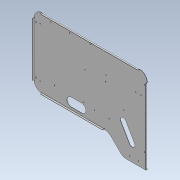
# Autodesk Inventor part: Монтажный лист
Saved by Autodesk Inventor 2021.2 (Build 252289000, 289)
## iProperties
Created: 2022-11-29
Part Number: Монтажный лист
Material: Типовые
Document SubType Name: ЛистМат
Designer: Voodoo
Density: 1 g/cm^3
Sheet Metal Rule: По умолчанию_мм
Appearance: По умолчанию
Mass: 97.8179 g
Surface Area: 1975.67 cm^2
Volume: 97.8179 cm^3
Flat Pattern Width: 29.2262 cm
Flat Pattern Length: 39.5524 cm
Flat Pattern Area: 1155.97 cm^2
Sheet Metal Width: 292,262 мм
Sheet Metal Length: 395,524 мм
Sheet Metal Area: 115596,583 мм^2
Author: Voodoo
Autodesk Inventor part; units mm, degrees
ref_plane "YZ Plane" through (0, 0, 0) normal (1, 0, 0) x (0, 1, 0)
ref_plane "XZ Plane" through (0, 0, 0) normal (0, 1, 0) x (-1, 0, 0)
ref_plane "XY Plane" through (0, 0, 0) normal (0, 0, 1) x (1, 0, 0)
sketch "Эскиз1" plane through (0, 0, 0) normal (0, 0, 1) x (1, 0, 0)
  line L0 (-166.5, -124) -> (46.0736, -124)
  line L1 (198.5, -124) -> (198.5, 92)
  line L2 (166.5, 124) -> (-166.5, 124)
  line L3 (-198.5, 92) -> (-198.5, -92)
  line L4 (-198.5, -124) -> (198.5, 124) construction
  line L5 (198.5, -124) -> (-198.5, 124) construction
  arc A0 (-166.5, 124) -> (-198.5, 92) centre (-166.5, 92) ccw
  arc A1 (198.5, 92) -> (166.5, 124) centre (166.5, 92) ccw
  arc A2 (-198.5, -92) -> (-166.5, -124) centre (-166.5, -92) ccw
  line L6 (198.5, -124) -> (198.5, -162)
  line L7 (186.5, -174) -> (120.9264, -174)
  line L8 (99.7132, -165.2132) -> (67.2868, -132.7868)
  arc A3 (186.5, -174) -> (198.5, -162) centre (186.5, -162) ccw
  arc A4 (99.7132, -165.2132) -> (120.9264, -174) centre (120.9264, -144) ccw
  arc A5 (67.2868, -132.7868) -> (46.0736, -124) centre (46.0736, -154) ccw
  line L9 (-166.5, 119) -> (166.5, 119)
  arc A6 (193.5, 92) -> (166.5, 119) centre (166.5, 92) ccw
  line L10 (193.5, 92) -> (193.5, -145)
  line L11 (193.5, -145) -> (193.5, -162)
  arc A7 (186.5, -169) -> (193.5, -162) centre (186.5, -162) ccw
  line L12 (186.5, -169) -> (120.9264, -169)
  arc A8 (103.2487, -161.6777) -> (120.9264, -169) centre (120.9264, -144) ccw
  line L13 (103.2487, -161.6777) -> (70.8223, -129.2513)
  arc A9 (70.8223, -129.2513) -> (46.0736, -119) centre (46.0736, -154) ccw
  line L14 (46.0736, -119) -> (-166.5, -119)
  arc A10 (-193.5, -92) -> (-166.5, -119) centre (-166.5, -92) ccw
  line L15 (-193.5, -92) -> (-193.5, 92)
  arc A11 (-166.5, 119) -> (-193.5, 92) centre (-166.5, 92) ccw
  point P0 (0, 0)
  point P1 (198.5, -174)
  point P2 (108.5, -174)
  dimension "d2" = 397
  dimension "d3" = 248
  dimension "d4" = 32
  dimension "d5" = 298
  dimension "d6" = 12
  dimension "d7" = 50
  dimension "d8" = 90
  dimension "d9" = 135
  dimension "d10" = 30
  dimension "d11" = 5
  constraints: 32 end point, 24 point on circle, 12 centre point, 12 point on line, 12 tangent, 4 parallel, 4 perpendicular, 3 equal radius, 2 midpoint, 1 horizontal, 12 other
  measures "d2" distance of L5.end L4.end
  measures "d3" distance of L4.end L1.start
  measures "d4" radius of A0
  measures "d5" distance between parallel lines of L7 L2
  measures "d6" radius of A3
  measures "d7" distance between parallel lines of L0 L7
  measures "d8" distance from line of L6 point (108.5, -174)
  measures "d9" angle of L0 L8
  measures "d10" radius of A4
  measures "d11" distance between parallel lines of L2 L9
extrude "Пластина1" add sketch "Эскиз1" along normal blind 1 contours L9 A6 L10 L11 A7 L12 A8 L13 A9 L14 A10 L15 A11
sketch "Эскиз4" plane through (-192.5, -92, 0) normal (-1, 0, 0) x (0, -1, 0)
  line L0 (-184, 0) -> (0, 0)
  line L1 (0, 0) -> (0, 6)
  line L2 (0, 6) -> (-184, 6)
  line L3 (-184, 6) -> (-184, 0)
  constraints: 6 end point, 1 horizontal, 1 perpendicular, 1 vertical
edge flange "Фланец1" height 6 angle 90 thickness 1 bend radius 1 thickness toward (-1, 0, 0) relief straight relief width 1 relief depth 0.5 corner gap 1 corner form 0 edges at (-193.5, 0, 1) (-60.2132, -119, 1) (0, 119, 1) (193.5, -26.5, 1) (193.5, -153.5, 1) wall of the first edge with corners at (-192.5, 92, 0) (-192.5, -92, 0) (-192.5, -92, 6) (-192.5, 92, 6)
bend "Сгиб1"
corner "УглСтык1"
sketch "Эскиз5" plane through (0, 0, 1) normal (0, 0, 1) x (1, 0, 0)
  arc A0 (-193.4815, -93) -> (-167.5, -118.9815) centre (-166.5, -92) ccw projected
  arc A1 (70.8223, -129.2513) -> (47.0736, -119.0143) centre (46.0736, -154) ccw projected
  line L0 (103.2487, -161.6777) -> (70.8223, -129.2513) projected
  arc A2 (103.2487, -161.6777) -> (120.9264, -169) centre (120.9264, -144) ccw projected
  line L1 (186.5, -169) -> (120.9264, -169) projected
  arc A3 (186.5, -169) -> (193.4282, -163) centre (186.5, -162) ccw projected
  arc A4 (193.4815, 93) -> (167.5, 118.9815) centre (166.5, 92) ccw projected
  arc A5 (-167.5, 118.9815) -> (-193.4815, 93) centre (-166.5, 92) ccw projected
  circle A6 centre (-186, 82) radius 2.5
  circle A7 centre (-186, -82) radius 2.5
  circle A8 centre (0, 111.1) radius 2.5
  circle A9 centre (185.8, 82) radius 2.5
  circle A10 centre (185.8, -116.8) radius 2.5
  line L2 (191, 93) -> (193.4815, 93) projected
  line L3 (167.5, 118.9815) -> (167.5, 116.5) projected
  line L4 (167.5, 116.5) -> (166.5, 116.5) projected
  line L5 (166.5, 116.5) -> (166.5, 117) projected
  line L6 (166.5, 117) -> (-166.5, 117) projected
  line L7 (-166.5, 117) -> (-166.5, 116.5) projected
  line L8 (-166.5, 116.5) -> (-167.5, 116.5) projected
  line L9 (-167.5, 116.5) -> (-167.5, 118.9815) projected
  line L10 (-193.4815, 93) -> (-191, 93) projected
  line L11 (-191, 93) -> (-191, 92) projected
  line L12 (-191, 92) -> (-191.5, 92) projected
  line L13 (-191.5, 92) -> (-191.5, -92) projected
  line L14 (-191.5, -92) -> (-191, -92) projected
  line L15 (-191, -92) -> (-191, -93) projected
  line L16 (-191, -93) -> (-193.4815, -93) projected
  line L17 (-167.5, -118.9815) -> (-167.5, -116.5) projected
  line L18 (-167.5, -116.5) -> (-166.5, -116.5) projected
  line L19 (-166.5, -116.5) -> (-166.5, -117) projected
  line L20 (-166.5, -117) -> (46.0736, -117) projected
  line L21 (46.0736, -117) -> (46.0736, -116.5) projected
  line L22 (46.0736, -116.5) -> (47.0736, -116.5) projected
  line L23 (47.0736, -116.5) -> (47.0736, -119.0143) projected
  line L24 (193.4282, -163) -> (191, -163) projected
  line L25 (191, -163) -> (191, -162) projected
  line L26 (191, -162) -> (191.5, -162) projected
  line L27 (191.5, -162) -> (191.5, 92) projected
  line L28 (191.5, 92) -> (191, 92) projected
  line L29 (191, 92) -> (191, 93) projected
  line L30 (166.5, 119) -> (-166.5, 119) projected
  line L31 (193.5, -162) -> (193.5, 92) projected
  line L32 (-193.5, 92) -> (-193.5, -92) projected
  line L33 (-166.5, -119) -> (46.0736, -119) projected
  point P0 (0, 0)
  point P1 (0, 119)
  dimension "d34" = 5
  dimension "d37" = 5
  dimension "d40" = 5
  dimension "d43" = 5
  dimension "d45" = 5
  dimension "d47" = 52.2
  dimension "d136" = 37
  dimension "d137" = 7.7
  dimension "d138" = 7.7
  dimension "d139" = 7.9
  dimension "d140" = 7.5
  dimension "d141" = 37
  dimension "d142" = 37
  dimension "d143" = 7.5
  constraints: 5 centre point, 1 midpoint, 1 vertical alignment
  measures "d34" diameter of A6
  measures "d37" diameter of A7
  measures "d40" diameter of A8
  measures "d43" diameter of A9
  measures "d45" diameter of A10
  measures "d47" distance from line of A10.centre L1
  measures "d136" distance from line of A9.centre L30
  measures "d137" distance from line of A10.centre L31
  measures "d138" distance from line of A9.centre L31
  measures "d139" distance from line of A8.centre L30
  measures "d140" distance from line of A6.centre L32
  measures "d141" distance from line of L30 A6.centre
  measures "d142" distance from line of L33 A7.centre
  measures "d143" distance from line of A7.centre L32
extrude "Вырез3" cut sketch "Эскиз5" against normal blind 1 contours A6 | A7 | A8 | A9 | A10
sketch "Эскиз6" plane through (0, 0, 1) normal (0, 0, 1) x (1, 0, 0)
  circle A0 centre (185.8, 82) radius 2.5 projected
  circle A1 centre (-186, -82) radius 2.5 projected
  circle A2 centre (-186, 82) radius 2.5 projected
  circle A3 centre (0, 111.1) radius 2.5 projected
  circle A4 centre (185.8, -116.8) radius 2.5 projected
  arc A5 (-193.4815, -93) -> (-167.5, -118.9815) centre (-166.5, -92) ccw projected
  arc A6 (70.8223, -129.2513) -> (47.0736, -119.0143) centre (46.0736, -154) ccw projected
  line L0 (103.2487, -161.6777) -> (70.8223, -129.2513) projected
  arc A7 (103.2487, -161.6777) -> (120.9264, -169) centre (120.9264, -144) ccw projected
  line L1 (186.5, -169) -> (120.9264, -169) projected
  arc A8 (186.5, -169) -> (193.4282, -163) centre (186.5, -162) ccw projected
  arc A9 (193.4815, 93) -> (167.5, 118.9815) centre (166.5, 92) ccw projected
  arc A10 (-167.5, 118.9815) -> (-193.4815, 93) centre (-166.5, 92) ccw projected
  circle A11 centre (-19.5, 24.5) radius 1.5
  circle A12 centre (51.5, 24.5) radius 1.5
  circle A13 centre (53, 44.5) radius 1.5
  circle A14 centre (154, 44.5) radius 1.5
  circle A15 centre (-135.8, 107) radius 1.5
  circle A16 centre (-71.5, 107) radius 1.5
  line L2 (191, 93) -> (193.4815, 93) projected
  line L3 (167.5, 118.9815) -> (167.5, 116.5) projected
  line L4 (167.5, 116.5) -> (166.5, 116.5) projected
  line L5 (166.5, 116.5) -> (166.5, 117) projected
  line L6 (166.5, 117) -> (-166.5, 117) projected
  line L7 (-166.5, 117) -> (-166.5, 116.5) projected
  line L8 (-166.5, 116.5) -> (-167.5, 116.5) projected
  line L9 (-167.5, 116.5) -> (-167.5, 118.9815) projected
  line L10 (-193.4815, 93) -> (-191, 93) projected
  line L11 (-191, 93) -> (-191, 92) projected
  line L12 (-191, 92) -> (-191.5, 92) projected
  line L13 (-191.5, 92) -> (-191.5, -92) projected
  line L14 (-191.5, -92) -> (-191, -92) projected
  line L15 (-191, -92) -> (-191, -93) projected
  line L16 (-191, -93) -> (-193.4815, -93) projected
  line L17 (-167.5, -118.9815) -> (-167.5, -116.5) projected
  line L18 (-167.5, -116.5) -> (-166.5, -116.5) projected
  line L19 (-166.5, -116.5) -> (-166.5, -117) projected
  line L20 (-166.5, -117) -> (46.0736, -117) projected
  line L21 (46.0736, -117) -> (46.0736, -116.5) projected
  line L22 (46.0736, -116.5) -> (47.0736, -116.5) projected
  line L23 (47.0736, -116.5) -> (47.0736, -119.0143) projected
  line L24 (193.4282, -163) -> (191, -163) projected
  line L25 (191, -163) -> (191, -162) projected
  line L26 (191, -162) -> (191.5, -162) projected
  line L27 (191.5, -162) -> (191.5, 92) projected
  line L28 (191.5, 92) -> (191, 92) projected
  line L29 (191, 92) -> (191, 93) projected
  line L30 (-193.5, 92) -> (-193.5, -92) projected
  line L31 (166.5, 119) -> (-166.5, 119) projected
  line L32 (193.5, -162) -> (193.5, 92) projected
  point P0 (0, 0)
  dimension "d51" = 3
  dimension "d52" = 3
  dimension "d53" = 3
  dimension "d54" = 3
  dimension "d56" = 71
  dimension "d58" = 101
  dimension "d61" = 3
  dimension "d62" = 3
  dimension "d63" = 64.3
  dimension "d123" = 74.5
  dimension "d124" = 39.5
  dimension "d125" = 142
  dimension "d126" = 20
  dimension "d127" = 12
  dimension "d128" = 122
  constraints: 6 centre point, 3 horizontal alignment
  measures "d51" diameter of A11
  measures "d52" diameter of A12
  measures "d53" diameter of A13
  measures "d54" diameter of A14
  measures "d56" distance of A12.centre A11.centre
  measures "d58" distance of A13.centre A14.centre
  measures "d61" diameter of A15
  measures "d62" diameter of A16
  measures "d63" distance of A16.centre A15.centre
  measures "d123" distance from line of L31 A14.centre
  measures "d124" distance from line of L32 A14.centre
  measures "d125" distance from line of L32 A12.centre
  measures "d126" vertical distance of A13.centre A12.centre
  measures "d127" distance from line of A16.centre L31
  measures "d128" distance from line of L30 A16.centre
extrude "Вырез4" cut sketch "Эскиз6" against normal blind 1 contours A11 | A12 | A13 | A14 | A15 | A16
sketch "Эскиз7" plane through (0, 0, 1) normal (0, 0, 1) x (1, 0, 0)
  circle A0 centre (-135.8, 107) radius 1.5 projected
  circle A1 centre (53, 44.5) radius 1.5 projected
  circle A2 centre (-19.5, 24.5) radius 1.5 projected
  circle A3 centre (51.5, 24.5) radius 1.5 projected
  circle A4 centre (154, 44.5) radius 1.5 projected
  circle A5 centre (-71.5, 107) radius 1.5 projected
  circle A6 centre (185.8, 82) radius 2.5 projected
  circle A7 centre (-186, -82) radius 2.5 projected
  circle A8 centre (-186, 82) radius 2.5 projected
  circle A9 centre (0, 111.1) radius 2.5 projected
  circle A10 centre (185.8, -116.8) radius 2.5 projected
  arc A11 (-193.4815, -93) -> (-167.5, -118.9815) centre (-166.5, -92) ccw projected
  arc A12 (70.8223, -129.2513) -> (47.0736, -119.0143) centre (46.0736, -154) ccw projected
  line L0 (103.2487, -161.6777) -> (70.8223, -129.2513) projected
  arc A13 (103.2487, -161.6777) -> (120.9264, -169) centre (120.9264, -144) ccw projected
  line L1 (186.5, -169) -> (120.9264, -169) projected
  arc A14 (186.5, -169) -> (193.4282, -163) centre (186.5, -162) ccw projected
  arc A15 (193.4815, 93) -> (167.5, 118.9815) centre (166.5, 92) ccw projected
  arc A16 (-167.5, 118.9815) -> (-193.4815, 93) centre (-166.5, 92) ccw projected
  circle A17 centre (-172.5, 84) radius 1.5
  circle A18 centre (-172.5, -86) radius 1.5
  circle A19 centre (172.5, 45) radius 1.5
  line L2 (0, 111.1) -> (0, 66.4707)
  line L3 (191, 93) -> (193.4815, 93) projected
  line L4 (167.5, 118.9815) -> (167.5, 116.5) projected
  line L5 (167.5, 116.5) -> (166.5, 116.5) projected
  line L6 (166.5, 116.5) -> (166.5, 117) projected
  line L7 (166.5, 117) -> (-166.5, 117) projected
  line L8 (-166.5, 117) -> (-166.5, 116.5) projected
  line L9 (-166.5, 116.5) -> (-167.5, 116.5) projected
  line L10 (-167.5, 116.5) -> (-167.5, 118.9815) projected
  line L11 (-193.4815, 93) -> (-191, 93) projected
  line L12 (-191, 93) -> (-191, 92) projected
  line L13 (-191, 92) -> (-191.5, 92) projected
  line L14 (-191.5, 92) -> (-191.5, -92) projected
  line L15 (-191.5, -92) -> (-191, -92) projected
  line L16 (-191, -92) -> (-191, -93) projected
  line L17 (-191, -93) -> (-193.4815, -93) projected
  line L18 (-167.5, -118.9815) -> (-167.5, -116.5) projected
  line L19 (-167.5, -116.5) -> (-166.5, -116.5) projected
  line L20 (-166.5, -116.5) -> (-166.5, -117) projected
  line L21 (-166.5, -117) -> (46.0736, -117) projected
  line L22 (46.0736, -117) -> (46.0736, -116.5) projected
  line L23 (46.0736, -116.5) -> (47.0736, -116.5) projected
  line L24 (47.0736, -116.5) -> (47.0736, -119.0143) projected
  line L25 (193.4282, -163) -> (191, -163) projected
  line L26 (191, -163) -> (191, -162) projected
  line L27 (191, -162) -> (191.5, -162) projected
  line L28 (191.5, -162) -> (191.5, 92) projected
  line L29 (191.5, 92) -> (191, 92) projected
  line L30 (191, 92) -> (191, 93) projected
  line L31 (166.5, 119) -> (-166.5, 119) projected
  point P0 (0, 0)
  dimension "d68" = 3
  dimension "d69" = 3
  dimension "d71" = 3
  dimension "d72" = 172.5
  dimension "d74" = 170
  dimension "d144" = 72
  dimension "d151" = 35
  dimension "d152" = 345
  constraints: 3 centre point, 2 end point, 1 vertical, 1 vertical alignment
  measures "d68" diameter of A17
  measures "d69" diameter of A18
  measures "d71" diameter of A19
  measures "d72" distance from line of A17.centre L2
  measures "d74" distance of A18.centre A17.centre
  measures "d144" distance from line of L7 A19.centre
  measures "d151" distance from line of A17.centre L31
  measures "d152" horizontal distance of A19.centre A17.centre
extrude "Вырез5" cut sketch "Эскиз7" against normal blind 1 contours A17 | A18 | A19
sketch "Эскиз8" plane through (0, 0, 0) normal (0, 0, -1) x (-1, 0, 0)
  circle A0 centre (135.8, 107) radius 1.5 projected
  circle A1 centre (-53, 44.5) radius 1.5 projected
  circle A2 centre (19.5, 24.5) radius 1.5 projected
  circle A3 centre (-51.5, 24.5) radius 1.5 projected
  circle A4 centre (-154, 44.5) radius 1.5 projected
  circle A5 centre (71.5, 107) radius 1.5 projected
  circle A6 centre (-185.8, 82) radius 2.5 projected
  circle A7 centre (186, -82) radius 2.5 projected
  circle A8 centre (186, 82) radius 2.5 projected
  circle A9 centre (0, 111.1) radius 2.5 projected
  circle A10 centre (-185.8, -116.8) radius 2.5 projected
  line L0 (-193.4815, 93) -> (-191, 93) projected
  line L1 (-191, 93) -> (-191, 92) projected
  line L2 (-191, 92) -> (-191.5, 92) projected
  line L3 (-191.5, 92) -> (-191.5, -162) projected
  line L4 (-191.5, -162) -> (-191, -162) projected
  line L5 (-191, -162) -> (-191, -163) projected
  line L6 (-191, -163) -> (-193.4282, -163) projected
  arc A11 (-193.4282, -163) -> (-186.5, -169) centre (-186.5, -162) ccw projected
  line L7 (-186.5, -169) -> (-120.9264, -169) projected
  arc A12 (-120.9264, -169) -> (-103.2487, -161.6777) centre (-120.9264, -144) ccw projected
  line L8 (-103.2487, -161.6777) -> (-70.8223, -129.2513) projected
  arc A13 (-47.0736, -119.0143) -> (-70.8223, -129.2513) centre (-46.0736, -154) ccw projected
  line L9 (-47.0736, -119.0143) -> (-47.0736, -116.5) projected
  line L10 (-47.0736, -116.5) -> (-46.0736, -116.5) projected
  line L11 (-46.0736, -116.5) -> (-46.0736, -117) projected
  line L12 (-46.0736, -117) -> (166.5, -117) projected
  line L13 (166.5, -117) -> (166.5, -116.5) projected
  line L14 (166.5, -116.5) -> (167.5, -116.5) projected
  line L15 (167.5, -116.5) -> (167.5, -118.9815) projected
  arc A14 (167.5, -118.9815) -> (193.4815, -93) centre (166.5, -92) ccw projected
  line L16 (193.4815, -93) -> (191, -93) projected
  line L17 (191, -93) -> (191, -92) projected
  line L18 (191, -92) -> (191.5, -92) projected
  line L19 (191.5, -92) -> (191.5, 92) projected
  line L20 (191.5, 92) -> (191, 92) projected
  line L21 (191, 92) -> (191, 93) projected
  line L22 (191, 93) -> (193.4815, 93) projected
  arc A15 (193.4815, 93) -> (167.5, 118.9815) centre (166.5, 92) ccw projected
  line L23 (167.5, 118.9815) -> (167.5, 116.5) projected
  line L24 (167.5, 116.5) -> (166.5, 116.5) projected
  line L25 (166.5, 116.5) -> (166.5, 117) projected
  line L26 (166.5, 117) -> (-166.5, 117) projected
  line L27 (-166.5, 117) -> (-166.5, 116.5) projected
  line L28 (-166.5, 116.5) -> (-167.5, 116.5) projected
  line L29 (-167.5, 116.5) -> (-167.5, 118.9815) projected
  arc A16 (-167.5, 118.9815) -> (-193.4815, 93) centre (-166.5, 92) ccw projected
  line L30 (-111.5, -62.0385) -> (-141.5, -114) construction
  line L31 (-120.1603, -57.0385) -> (-150.1603, -109)
  line L32 (-132.8397, -119) -> (-102.8397, -67.0385)
  arc A17 (-102.8397, -67.0385) -> (-120.1603, -57.0385) centre (-111.5, -62.0385) ccw
  arc A18 (-150.1603, -109) -> (-132.8397, -119) centre (-141.5, -114) ccw
  point P0 (0, 0)
  point P1 (-126.5, -88.0192)
  dimension "d80" = 20
  dimension "d81" = 60
  dimension "d84" = 30
  dimension "d153" = 50
  dimension "d154" = 55
  constraints: 8 end point, 4 point on circle, 4 tangent, 2 centre point, 1 midpoint, 1 parallel
  measures "d80" diameter of A18
  measures "d81" angle of L12 L30
  measures "d84" horizontal distance of L30.end L30.start
  measures "d153" distance from line of L3 L30.end
  measures "d154" distance from line of L7 L30.end
extrude "Вырез6" cut sketch "Эскиз8" against normal blind 1 contours A17 L32 A18 L31
sketch "Эскиз9" plane through (0, 0, 0) normal (0, 0, -1) x (-1, 0, 0)
  arc A0 (-150.1603, -109) -> (-132.8397, -119) centre (-141.5, -114) ccw projected
  line L0 (-150.1603, -109) -> (-120.1603, -57.0385) projected
  arc A1 (-102.8397, -67.0385) -> (-120.1603, -57.0385) centre (-111.5, -62.0385) ccw projected
  line L1 (-102.8397, -67.0385) -> (-132.8397, -119) projected
  circle A2 centre (135.8, 107) radius 1.5 projected
  circle A3 centre (-53, 44.5) radius 1.5 projected
  circle A4 centre (19.5, 24.5) radius 1.5 projected
  circle A5 centre (-51.5, 24.5) radius 1.5 projected
  circle A6 centre (-154, 44.5) radius 1.5 projected
  circle A7 centre (71.5, 107) radius 1.5 projected
  circle A8 centre (-185.8, 82) radius 2.5 projected
  circle A9 centre (186, -82) radius 2.5 projected
  circle A10 centre (186, 82) radius 2.5 projected
  circle A11 centre (0, 111.1) radius 2.5 projected
  circle A12 centre (-185.8, -116.8) radius 2.5 projected
  line L2 (-193.4815, 93) -> (-191, 93) projected
  line L3 (-191, 93) -> (-191, 92) projected
  line L4 (-191, 92) -> (-191.5, 92) projected
  line L5 (-191.5, 92) -> (-191.5, -162) projected
  line L6 (-191.5, -162) -> (-191, -162) projected
  line L7 (-191, -162) -> (-191, -163) projected
  line L8 (-191, -163) -> (-193.4282, -163) projected
  arc A13 (-193.4282, -163) -> (-186.5, -169) centre (-186.5, -162) ccw projected
  line L9 (-186.5, -169) -> (-120.9264, -169) projected
  arc A14 (-120.9264, -169) -> (-103.2487, -161.6777) centre (-120.9264, -144) ccw projected
  line L10 (-103.2487, -161.6777) -> (-70.8223, -129.2513) projected
  arc A15 (-47.0736, -119.0143) -> (-70.8223, -129.2513) centre (-46.0736, -154) ccw projected
  line L11 (-47.0736, -119.0143) -> (-47.0736, -116.5) projected
  line L12 (-47.0736, -116.5) -> (-46.0736, -116.5) projected
  line L13 (-46.0736, -116.5) -> (-46.0736, -117) projected
  line L14 (-46.0736, -117) -> (166.5, -117) projected
  line L15 (166.5, -117) -> (166.5, -116.5) projected
  line L16 (166.5, -116.5) -> (167.5, -116.5) projected
  line L17 (167.5, -116.5) -> (167.5, -118.9815) projected
  arc A16 (167.5, -118.9815) -> (193.4815, -93) centre (166.5, -92) ccw projected
  line L18 (193.4815, -93) -> (191, -93) projected
  line L19 (191, -93) -> (191, -92) projected
  line L20 (191, -92) -> (191.5, -92) projected
  line L21 (191.5, -92) -> (191.5, 92) projected
  line L22 (191.5, 92) -> (191, 92) projected
  line L23 (191, 92) -> (191, 93) projected
  line L24 (191, 93) -> (193.4815, 93) projected
  arc A17 (193.4815, 93) -> (167.5, 118.9815) centre (166.5, 92) ccw projected
  line L25 (167.5, 118.9815) -> (167.5, 116.5) projected
  line L26 (167.5, 116.5) -> (166.5, 116.5) projected
  line L27 (166.5, 116.5) -> (166.5, 117) projected
  line L28 (166.5, 117) -> (-166.5, 117) projected
  line L29 (-166.5, 117) -> (-166.5, 116.5) projected
  line L30 (-166.5, 116.5) -> (-167.5, 116.5) projected
  line L31 (-167.5, 116.5) -> (-167.5, 118.9815) projected
  arc A18 (-167.5, 118.9815) -> (-193.4815, 93) centre (-166.5, 92) ccw projected
  circle A19 centre (-113.5, -29) radius 1.5
  circle A20 centre (-13.5, -79) radius 1.5
  circle A21 centre (-63.5, -79) radius 1.5
  point P0 (0, 0)
  dimension "d87" = 3
  dimension "d88" = 3
  dimension "d89" = 3
  dimension "d145" = 140
  dimension "d146" = 78
  dimension "d147" = 50
  dimension "d148" = 50
  dimension "d149" = 50
  constraints: 3 centre point, 1 horizontal alignment
  measures "d87" diameter of A19
  measures "d88" diameter of A20
  measures "d89" diameter of A21
  measures "d145" distance from line of L9 A19.centre
  measures "d146" distance from line of L5 A19.centre
  measures "d147" horizontal distance of A21.centre A19.centre
  measures "d148" horizontal distance of A19.centre A21.centre
  measures "d149" distance of A21.centre A20.centre
extrude "Вырез7" cut sketch "Эскиз9" against normal blind 1 contours A19 | A20 | A21
sketch "Эскиз10" plane through (0, 0, 0) normal (0, 0, -1) x (-1, 0, 0)
  circle A0 centre (-13.5, -79) radius 1.5 projected
  circle A1 centre (-113.5, -29) radius 1.5 projected
  circle A2 centre (-63.5, -79) radius 1.5 projected
  arc A3 (-150.1603, -109) -> (-132.8397, -119) centre (-141.5, -114) ccw projected
  line L0 (-150.1603, -109) -> (-120.1603, -57.0385) projected
  arc A4 (-102.8397, -67.0385) -> (-120.1603, -57.0385) centre (-111.5, -62.0385) ccw projected
  line L1 (-102.8397, -67.0385) -> (-132.8397, -119) projected
  circle A5 centre (135.8, 107) radius 1.5 projected
  circle A6 centre (-53, 44.5) radius 1.5 projected
  circle A7 centre (19.5, 24.5) radius 1.5 projected
  circle A8 centre (-51.5, 24.5) radius 1.5 projected
  circle A9 centre (-154, 44.5) radius 1.5 projected
  circle A10 centre (71.5, 107) radius 1.5 projected
  circle A11 centre (-185.8, 82) radius 2.5 projected
  circle A12 centre (186, -82) radius 2.5 projected
  circle A13 centre (186, 82) radius 2.5 projected
  circle A14 centre (0, 111.1) radius 2.5 projected
  circle A15 centre (-185.8, -116.8) radius 2.5 projected
  line L2 (-193.4815, 93) -> (-191, 93) projected
  line L3 (-191, 93) -> (-191, 92) projected
  line L4 (-191, 92) -> (-191.5, 92) projected
  line L5 (-191.5, 92) -> (-191.5, -162) projected
  line L6 (-191.5, -162) -> (-191, -162) projected
  line L7 (-191, -162) -> (-191, -163) projected
  line L8 (-191, -163) -> (-193.4282, -163) projected
  arc A16 (-193.4282, -163) -> (-186.5, -169) centre (-186.5, -162) ccw projected
  line L9 (-186.5, -169) -> (-120.9264, -169) projected
  arc A17 (-120.9264, -169) -> (-103.2487, -161.6777) centre (-120.9264, -144) ccw projected
  line L10 (-103.2487, -161.6777) -> (-70.8223, -129.2513) projected
  arc A18 (-47.0736, -119.0143) -> (-70.8223, -129.2513) centre (-46.0736, -154) ccw projected
  line L11 (-47.0736, -119.0143) -> (-47.0736, -116.5) projected
  line L12 (-47.0736, -116.5) -> (-46.0736, -116.5) projected
  line L13 (-46.0736, -116.5) -> (-46.0736, -117) projected
  line L14 (-46.0736, -117) -> (166.5, -117) projected
  line L15 (166.5, -117) -> (166.5, -116.5) projected
  line L16 (166.5, -116.5) -> (167.5, -116.5) projected
  line L17 (167.5, -116.5) -> (167.5, -118.9815) projected
  arc A19 (167.5, -118.9815) -> (193.4815, -93) centre (166.5, -92) ccw projected
  line L18 (193.4815, -93) -> (191, -93) projected
  line L19 (191, -93) -> (191, -92) projected
  line L20 (191, -92) -> (191.5, -92) projected
  line L21 (191.5, -92) -> (191.5, 92) projected
  line L22 (191.5, 92) -> (191, 92) projected
  line L23 (191, 92) -> (191, 93) projected
  line L24 (191, 93) -> (193.4815, 93) projected
  arc A20 (193.4815, 93) -> (167.5, 118.9815) centre (166.5, 92) ccw projected
  line L25 (167.5, 118.9815) -> (167.5, 116.5) projected
  line L26 (167.5, 116.5) -> (166.5, 116.5) projected
  line L27 (166.5, 116.5) -> (166.5, 117) projected
  line L28 (166.5, 117) -> (-166.5, 117) projected
  line L29 (-166.5, 117) -> (-166.5, 116.5) projected
  line L30 (-166.5, 116.5) -> (-167.5, 116.5) projected
  line L31 (-167.5, 116.5) -> (-167.5, 118.9815) projected
  arc A21 (-167.5, 118.9815) -> (-193.4815, 93) centre (-166.5, 92) ccw projected
  line L32 (31, -95) -> (66, -95) construction
  line L33 (31, -80) -> (66, -80)
  line L34 (66, -110) -> (31, -110)
  arc A22 (31, -80) -> (31, -110) centre (31, -95) ccw
  arc A23 (66, -110) -> (66, -80) centre (66, -95) ccw
  point P0 (0, 0)
  point P1 (48.5, -95)
  dimension "d97" = 7
  dimension "d98" = 35
  dimension "d99" = 30
  dimension "d100" = 143
  constraints: 8 end point, 4 point on circle, 4 tangent, 2 centre point, 1 horizontal, 1 midpoint, 1 parallel
  measures "d97" distance between parallel lines of L34 L14
  measures "d98" distance of L32.start L32.end
  measures "d99" distance between parallel lines of L34 L33
  measures "d100" distance from line of L21 point (48.5, -95)
extrude "Вырез8" cut sketch "Эскиз10" against normal blind 1 contours L33 A23 L34 A22
sketch "Эскиз11" plane through (0, 0, 0) normal (0, 0, -1) x (-1, 0, 0)
  arc A0 (31, -80) -> (31, -110) centre (31, -95) ccw projected
  line L0 (31, -80) -> (66, -80) projected
  arc A1 (66, -110) -> (66, -80) centre (66, -95) ccw projected
  line L1 (66, -110) -> (31, -110) projected
  circle A2 centre (-13.5, -79) radius 1.5 projected
  circle A3 centre (-113.5, -29) radius 1.5 projected
  circle A4 centre (-63.5, -79) radius 1.5 projected
  arc A5 (-150.1603, -109) -> (-132.8397, -119) centre (-141.5, -114) ccw projected
  line L2 (-150.1603, -109) -> (-120.1603, -57.0385) projected
  arc A6 (-102.8397, -67.0385) -> (-120.1603, -57.0385) centre (-111.5, -62.0385) ccw projected
  line L3 (-102.8397, -67.0385) -> (-132.8397, -119) projected
  circle A7 centre (135.8, 107) radius 1.5 projected
  circle A8 centre (-53, 44.5) radius 1.5 projected
  circle A9 centre (19.5, 24.5) radius 1.5 projected
  circle A10 centre (-51.5, 24.5) radius 1.5 projected
  circle A11 centre (-154, 44.5) radius 1.5 projected
  circle A12 centre (71.5, 107) radius 1.5 projected
  circle A13 centre (-185.8, 82) radius 2.5 projected
  circle A14 centre (186, -82) radius 2.5 projected
  circle A15 centre (186, 82) radius 2.5 projected
  circle A16 centre (0, 111.1) radius 2.5 projected
  circle A17 centre (-185.8, -116.8) radius 2.5 projected
  line L4 (-193.4815, 93) -> (-191, 93) projected
  line L5 (-191, 93) -> (-191, 92) projected
  line L6 (-191, 92) -> (-191.5, 92) projected
  line L7 (-191.5, 92) -> (-191.5, -162) projected
  line L8 (-191.5, -162) -> (-191, -162) projected
  line L9 (-191, -162) -> (-191, -163) projected
  line L10 (-191, -163) -> (-193.4282, -163) projected
  arc A18 (-193.4282, -163) -> (-186.5, -169) centre (-186.5, -162) ccw projected
  line L11 (-186.5, -169) -> (-120.9264, -169) projected
  arc A19 (-120.9264, -169) -> (-103.2487, -161.6777) centre (-120.9264, -144) ccw projected
  line L12 (-103.2487, -161.6777) -> (-70.8223, -129.2513) projected
  arc A20 (-47.0736, -119.0143) -> (-70.8223, -129.2513) centre (-46.0736, -154) ccw projected
  line L13 (-47.0736, -119.0143) -> (-47.0736, -116.5) projected
  line L14 (-47.0736, -116.5) -> (-46.0736, -116.5) projected
  line L15 (-46.0736, -116.5) -> (-46.0736, -117) projected
  line L16 (-46.0736, -117) -> (166.5, -117) projected
  line L17 (166.5, -117) -> (166.5, -116.5) projected
  line L18 (166.5, -116.5) -> (167.5, -116.5) projected
  line L19 (167.5, -116.5) -> (167.5, -118.9815) projected
  arc A21 (167.5, -118.9815) -> (193.4815, -93) centre (166.5, -92) ccw projected
  line L20 (193.4815, -93) -> (191, -93) projected
  line L21 (191, -93) -> (191, -92) projected
  line L22 (191, -92) -> (191.5, -92) projected
  line L23 (191.5, -92) -> (191.5, 92) projected
  line L24 (191.5, 92) -> (191, 92) projected
  line L25 (191, 92) -> (191, 93) projected
  line L26 (191, 93) -> (193.4815, 93) projected
  arc A22 (193.4815, 93) -> (167.5, 118.9815) centre (166.5, 92) ccw projected
  line L27 (167.5, 118.9815) -> (167.5, 116.5) projected
  line L28 (167.5, 116.5) -> (166.5, 116.5) projected
  line L29 (166.5, 116.5) -> (166.5, 117) projected
  line L30 (166.5, 117) -> (-166.5, 117) projected
  line L31 (-166.5, 117) -> (-166.5, 116.5) projected
  line L32 (-166.5, 116.5) -> (-167.5, 116.5) projected
  line L33 (-167.5, 116.5) -> (-167.5, 118.9815) projected
  arc A23 (-167.5, 118.9815) -> (-193.4815, 93) centre (-166.5, 92) ccw projected
  circle A24 centre (23.5, -74) radius 1.5
  circle A25 centre (123.5, -74) radius 1.5
  line L34 (48.5, -80) -> (48.5, -99.1978) construction
  line L35 (166.5, -119) -> (-46.0736, -119) projected
  point P0 (0, 0)
  dimension "d114" = 3
  dimension "d115" = 3
  dimension "d116" = 25
  dimension "d117" = 75
  dimension "d118" = 45
  constraints: 2 centre point, 2 end point, 1 horizontal alignment, 1 midpoint, 1 vertical
  measures "d114" diameter of A24
  measures "d115" diameter of A25
  measures "d116" distance from line of A24.centre L34
  measures "d117" distance from line of L34 A25.centre
  measures "d118" distance from line of A24.centre L35
extrude "Вырез9" cut sketch "Эскиз11" against normal blind 1 contours A24 | A25
sketch "Эскиз14" plane through (0, 0, 0) normal (0, 0, -1) x (-1, 0, 0)
  circle A0 centre (23.5, -74) radius 1.5 projected
  circle A1 centre (123.5, -74) radius 1.5 projected
  arc A2 (31, -80) -> (31, -110) centre (31, -95) ccw projected
  line L0 (31, -80) -> (66, -80) projected
  arc A3 (66, -110) -> (66, -80) centre (66, -95) ccw projected
  line L1 (66, -110) -> (31, -110) projected
  circle A4 centre (-13.5, -79) radius 1.5 projected
  circle A5 centre (-113.5, -29) radius 1.5 projected
  circle A6 centre (-63.5, -79) radius 1.5 projected
  arc A7 (-150.1603, -109) -> (-132.8397, -119) centre (-141.5, -114) ccw projected
  line L2 (-150.1603, -109) -> (-120.1603, -57.0385) projected
  arc A8 (-102.8397, -67.0385) -> (-120.1603, -57.0385) centre (-111.5, -62.0385) ccw projected
  line L3 (-102.8397, -67.0385) -> (-132.8397, -119) projected
  circle A9 centre (172.5, -86) radius 1.5 projected
  circle A10 centre (172.5, 84) radius 1.5 projected
  circle A11 centre (-172.5, 45) radius 1.5 projected
  circle A12 centre (135.8, 107) radius 1.5 projected
  circle A13 centre (-53, 44.5) radius 1.5 projected
  circle A14 centre (19.5, 24.5) radius 1.5 projected
  circle A15 centre (-51.5, 24.5) radius 1.5 projected
  circle A16 centre (-154, 44.5) radius 1.5 projected
  circle A17 centre (71.5, 107) radius 1.5 projected
  circle A18 centre (-185.8, 82) radius 2.5 projected
  circle A19 centre (186, -82) radius 2.5 projected
  circle A20 centre (186, 82) radius 2.5 projected
  circle A21 centre (0, 111.1) radius 2.5 projected
  circle A22 centre (-185.8, -116.8) radius 2.5 projected
  line L4 (-193.4815, 93) -> (-191, 93) projected
  line L5 (-191, 93) -> (-191, 92) projected
  line L6 (-191, 92) -> (-191.5, 92) projected
  line L7 (-191.5, 92) -> (-191.5, -162) projected
  line L8 (-191.5, -162) -> (-191, -162) projected
  line L9 (-191, -162) -> (-191, -163) projected
  line L10 (-191, -163) -> (-193.4282, -163) projected
  arc A23 (-193.4282, -163) -> (-186.5, -169) centre (-186.5, -162) ccw projected
  line L11 (-186.5, -169) -> (-120.9264, -169) projected
  arc A24 (-120.9264, -169) -> (-103.2487, -161.6777) centre (-120.9264, -144) ccw projected
  line L12 (-103.2487, -161.6777) -> (-70.8223, -129.2513) projected
  arc A25 (-47.0736, -119.0143) -> (-70.8223, -129.2513) centre (-46.0736, -154) ccw projected
  line L13 (-47.0736, -119.0143) -> (-47.0736, -116.5) projected
  line L14 (-47.0736, -116.5) -> (-46.0736, -116.5) projected
  line L15 (-46.0736, -116.5) -> (-46.0736, -117) projected
  line L16 (-46.0736, -117) -> (166.5, -117) projected
  line L17 (166.5, -117) -> (166.5, -116.5) projected
  line L18 (166.5, -116.5) -> (167.5, -116.5) projected
  line L19 (167.5, -116.5) -> (167.5, -118.9815) projected
  arc A26 (167.5, -118.9815) -> (193.4815, -93) centre (166.5, -92) ccw projected
  line L20 (193.4815, -93) -> (191, -93) projected
  line L21 (191, -93) -> (191, -92) projected
  line L22 (191, -92) -> (191.5, -92) projected
  line L23 (191.5, -92) -> (191.5, 92) projected
  line L24 (191.5, 92) -> (191, 92) projected
  line L25 (191, 92) -> (191, 93) projected
  line L26 (191, 93) -> (193.4815, 93) projected
  arc A27 (193.4815, 93) -> (167.5, 118.9815) centre (166.5, 92) ccw projected
  line L27 (167.5, 118.9815) -> (167.5, 116.5) projected
  line L28 (167.5, 116.5) -> (166.5, 116.5) projected
  line L29 (166.5, 116.5) -> (166.5, 117) projected
  line L30 (166.5, 117) -> (-166.5, 117) projected
  line L31 (-166.5, 117) -> (-166.5, 116.5) projected
  line L32 (-166.5, 116.5) -> (-167.5, 116.5) projected
  line L33 (-167.5, 116.5) -> (-167.5, 118.9815) projected
  arc A28 (-167.5, 118.9815) -> (-193.4815, 93) centre (-166.5, 92) ccw projected
  circle A29 centre (-163.5, -154) radius 1.5
  circle A30 centre (-133.5, -154) radius 1.5
  line L34 (-193.5, -162) -> (-193.5, 92) projected
  point P0 (0, 0)
  dimension "d155" = 3
  dimension "d156" = 3
  dimension "d157" = 15
  dimension "d158" = 15
  dimension "d159" = 30
  dimension "d160" = 30
  constraints: 2 centre point
  measures "d155" diameter of A29
  measures "d156" diameter of A30
  measures "d157" distance from line of A29.centre L11
  measures "d158" distance from line of L11 A30.centre
  measures "d159" distance of A30.centre A29.centre
  measures "d160" distance from line of A29.centre L34
extrude "Вырез11" cut sketch "Эскиз14" against normal blind 1 contours A29 | A30
equation "\"d49\" = Толщина"
equation "\"d66\" = Толщина"
equation "\"d68\" = d69"
equation "\"d69\" = d70"
equation "\"d76\" = Толщина"
equation "\"d85\" = Толщина"
equation "\"d95\" = Толщина"
equation "\"d101\" = Толщина"
equation "\"d119\" = Толщина"
equation "\"d12\" = Толщина"
equation "\"d24\" = Ширина_просечки"
equation "\"d25\" = Глубина_просечки"
equation "\"d26\" = Мин_остаток"
equation "\"d27\" = Радиус_перехода"
equation "\"d30\" = Радиус_гибки"
equation "\"d31\" = Размер_просечки"
equation "\"d32\" = Размер_зазора"
equation "\"d33\" = Радиус_Якоби"
equation "\"Радиус_гибки\" = Толщина"
equation "\"Ширина_просечки\" = Толщина"
equation "\"Глубина_просечки\" = 0.5 * Толщина"
equation "\"Размер_просечки\" = 4 * Толщина"
equation "\"Мин_остаток\" = 2 * Толщина"
equation "\"Радиус_перехода\" = Радиус_гибки"
equation "\"Радиус_Якоби\" = Радиус_гибки"
equation "\"Размер_зазора\" = Толщина"
equation "\"d70\" = d71"
equation "\"Толщина\" = 1"
